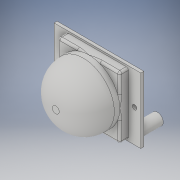
# Autodesk Inventor part: PIR_Sensor
Saved by Autodesk Inventor 2017 (Build 210142000, 142)
## iProperties
Created: 2018-02-28
Part Number: PIR_Sensor
Material: Generic
Document SubType Name: Modeling
Designer: Mitch
Density: 1 g/cm^3
Appearance: Default
Author: Mitch
Autodesk Inventor part; units mm, degrees
ref_plane "YZ Plane" through (0, 0, 0) normal (1, 0, 0) x (0, 1, 0)
ref_plane "XZ Plane" through (0, 0, 0) normal (0, 1, 0) x (-1, 0, 0)
ref_plane "XY Plane" through (0, 0, 0) normal (0, 0, 1) x (1, 0, 0)
sketch "Sketch1" plane through (0, 0, 0) normal (0, 0, 1) x (1, 0, 0)
  line L0 (0, 0) -> (32.004, 0)
  line L1 (32.004, 0) -> (32.004, 24.13)
  line L2 (32.004, 24.13) -> (0, 24.13)
  line L3 (0, 24.13) -> (0, 0)
  dimension "d0" = 32.004
  dimension "d1" = 24.13
  constraints: 8 end point, 2 parallel, 1 horizontal, 1 perpendicular
  measures "d0" distance of L2.end L1.end
  measures "d1" distance of L1.end L0.end
extrude "Extrusion1" add sketch "Sketch1" along normal blind 1.143
sketch "Sketch2" plane through (0, 0, 1.143) normal (0, 0, 1) x (1, 0, 0)
  line L0 (32.004, 24.13) -> (0, 24.13) projected
  line L1 (0, 0) -> (32.004, 0) projected
  line L2 (27.432, 23.495) -> (4.572, 23.495)
  line L3 (4.572, 0.635) -> (27.432, 0.635)
  line L4 (0, 24.13) -> (0, 0) projected
  line L5 (4.572, 0.635) -> (4.572, 23.495)
  line L6 (32.004, 0) -> (32.004, 24.13) projected
  line L7 (4.572, 19.558) -> (4.572, 4.572)
  line L8 (27.432, 0.635) -> (27.432, 23.495)
  dimension "d4" = 0.635
  dimension "d5" = 0.635
  dimension "d6" = 4.572
  dimension "d7" = 4.572
  constraints: 10 end point, 2 parallel
  measures "d4" distance between parallel lines of L0 L2
  measures "d5" distance between parallel lines of L1 L3
  measures "d6" distance between parallel lines of L4 L5
  measures "d7" distance between parallel lines of L6 L8
extrude "Extrusion2" add sketch "Sketch2" along normal blind 3.175 contours L8 L3 L5 L2
sketch "Sketch3" plane through (0, 0, 4.318) normal (0, 0, 1) x (1, 0, 0)
  line L0 (4.572, 0.635) -> (27.432, 0.635) projected
  line L1 (4.572, 0.635) -> (27.432, 23.495)
  circle A0 centre (16.002, 12.065) radius 11.43
  point P0 (0, 0)
  constraints: 2 end point, 1 centre point, 1 midpoint
extrude "Extrusion3" add sketch "Sketch3" along normal blind 12.192 contours A0 L1 | A0 L1
fillet "Fillet1" radius 10.16 1 edges at (4.572, 12.065, 16.51)
fillet "Fillet2" radius 0.7937 12 edges at (27.432, 23.495, 2.7305) (27.432, 17.78, 4.318) (21.717, 23.495, 4.318) (27.432, 6.35, 4.318) (21.717, 0.635, 4.318) (27.432, 0.635, 2.7305) (10.287, 0.635, 4.318) (4.572, 6.35, 4.318) (4.572, 0.635, 2.7305) (4.572, 23.495, 2.7305) (10.287, 23.495, 4.318) (4.572, 17.78, 4.318)
hole "Hole1" at (29.718, 12.065, 1.143) direction (0, 0, -1) diameter 1.6764 depth 25.4 tip angle 118
hole "Hole2" at (2.286, 12.065, 1.143) direction (0, 0, -1) diameter 1.6764 depth 25.4 tip angle 118
sketch "Sketch4" plane through (0, 0, 0) normal (0, 0, -1) x (-1, 0, 0)
  circle A0 centre (-28.2603, 2.6421) radius 2.1209
  point P0 (0, 0)
  dimension "d32" = 4.2418
  constraints: 1 centre point
  measures "d32" diameter of A0
extrude "Extrusion4" add sketch "Sketch4" along normal blind 8.763
body "Solid1"
